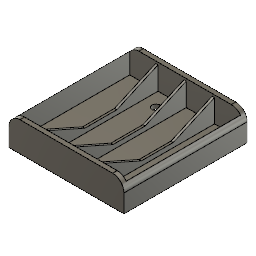
Fusion360_BatteryBox_AAA4 (Autodesk Fusion 360 design; units mm, degrees)
Autodesk Fusion 360 part; units mm, degrees
sketch "スケッチ1" plane through (0, 0, 0) normal (0, 1, 0) x (1, 0, 0)
  line L0 (25.25, -27) -> (-25.25, -27)
  line L1 (-25.25, -27) -> (-25.25, 27)
  line L2 (-25.25, 27) -> (25.25, 27)
  line L3 (25.25, 27) -> (25.25, -27)
  line L4 (25.25, -27) -> (-25.25, 27) construction
  line L5 (-25.25, -27) -> (25.25, 27) construction
  dimension "d1" = 50.5
  dimension "d2" = 54
sketch "スケッチ2" plane through (12.875, 0, 0) normal (1, 0, 0) x (0, 0, -1)
  line L0 (-25, 2) -> (25, 2)
  line L1 (25, 2) -> (25, 12)
  line L2 (25, 12) -> (-25, 12)
  line L3 (-25, 12) -> (-25, 2)
  line L4 (25, 2) -> (7, 2) construction
  line L5 (7, 2) -> (7, 4) construction
  line L6 (7, 4) -> (25, 4) construction
  line L7 (25, 4) -> (25, 2) construction
  line L8 (7, 4) -> (-7, 4)
  line L9 (-7, 4) -> (-7, 12)
  line L10 (-7, 12) -> (7, 12)
  line L11 (7, 12) -> (7, 4)
  dimension "d7" = 18
  dimension "d8" = 2
  dimension "d11" = 14
sketch "スケッチ3" plane through (0, 2, 0) normal (0, 1, 0) x (-1, 0, 0)
  circle A0 centre (-6.1875, 18.4923) radius 1.75
  line L0 (-0.5, -25) -> (-0.5, 25)
  line L1 (-0.5, 25) -> (-11.875, 25)
  line L2 (-11.875, 25) -> (-11.875, -25)
  line L3 (-11.875, -25) -> (-0.5, -25)
  line L4 (-6.1875, 18.4923) -> (6.1875, 18.4923) construction
  line L5 (6.1875, 18.4923) -> (6.1875, -18.4923) construction
  line L6 (6.1875, -18.4923) -> (-6.1875, -18.4923) construction
  line L7 (-6.1875, -18.4923) -> (-6.1875, 18.4923) construction
  circle A1 centre (6.1875, -18.4923) radius 1.75
  dimension "d12" = 12.375
  dimension "d13" = 36.9846
  dimension "d14" = 3.5
  measures "d14" diameter of A1
sketch "スケッチ4" plane through (0, 2, 0) normal (0, 1, 0) x (-1, 0, 0)
  line L0 (-0.5, -25) -> (-0.5, 25)
  line L1 (-0.5, 25) -> (-11.875, 25)
  line L2 (-11.875, 25) -> (-11.875, -25)
  line L3 (-11.875, -25) -> (-0.5, -25)
  line L4 (-11.875, 25) -> (-6.1875, 25) construction
  line L5 (-6.1875, 25) -> (-6.1875, 18.4923) construction
  line L6 (-6.1875, 18.4923) -> (-11.875, 18.4923) construction
  line L7 (-11.875, 18.4923) -> (-11.875, 25) construction
  circle A0 centre (-6.1875, 18.4923) radius 1.75
  dimension "d17" = 5.6875
  dimension "d18" = 6.5077
  dimension "d19" = 3.5
  measures "d19" diameter of A0
sketch "スケッチ5" plane through (0, 2, 0) normal (0, 1, 0) x (-1, 0, 0)
  line L0 (0.5, 25) -> (0.5, -25)
  line L1 (0.5, -25) -> (24.25, -25)
  line L2 (24.25, -25) -> (24.25, 25)
  line L3 (24.25, 25) -> (0.5, 25)
  line L4 (0.5, -25) -> (11.875, -25) construction
  line L5 (11.875, -25) -> (11.875, 25) construction
  line L6 (11.875, 25) -> (0.5, 25) construction
  line L7 (0.5, 25) -> (0.5, -25) construction
  line L8 (11.875, -25) -> (12.875, -25)
  line L9 (12.875, -25) -> (12.875, 25)
  line L10 (12.875, 25) -> (11.875, 25)
  line L11 (11.875, 25) -> (11.875, -25)
  dimension "d20" = 50
  dimension "d23" = 11.375
  dimension "d24" = 1
  dimension "d25" = 50
  measures "d23" distance of origin
sketch "スケッチ6" plane through (0, 2, 0) normal (0, 1, 0) x (-1, 0, 0)
  line L0 (-11.875, 25) -> (-11.875, -25)
  line L1 (-11.875, -25) -> (24.25, -25)
  line L2 (24.25, -25) -> (24.25, 25)
  line L3 (24.25, 25) -> (-11.875, 25)
  line L4 (-11.875, -25) -> (-0.5, -25) construction
  line L5 (-0.5, -25) -> (-0.5, 25) construction
  line L6 (-0.5, 25) -> (-11.875, 25) construction
  line L7 (-11.875, 25) -> (-11.875, -25) construction
  line L8 (-0.5, -25) -> (0.5, -25)
  line L9 (0.5, -25) -> (0.5, 25)
  line L10 (0.5, 25) -> (-0.5, 25)
  line L11 (-0.5, 25) -> (-0.5, -25)
  dimension "d26" = 11.375
  dimension "d29" = 50
  dimension "d30" = 50
  dimension "d31" = 1
  measures "d26" distance of origin
sketch "スケッチ7" plane through (0, 2, 0) normal (0, 1, 0) x (-1, 0, 0)
  line L0 (-24.25, -25) -> (24.25, -25)
  line L1 (24.25, -25) -> (24.25, 25)
  line L2 (24.25, 25) -> (-24.25, 25)
  line L3 (-24.25, 25) -> (-24.25, -25)
  line L4 (-24.25, -25) -> (-12.875, -25) construction
  line L5 (-12.875, -25) -> (-12.875, 25) construction
  line L6 (-12.875, 25) -> (-24.25, 25) construction
  line L7 (-24.25, 25) -> (-24.25, -25) construction
  line L8 (-12.875, -25) -> (-11.875, -25)
  line L9 (-11.875, -25) -> (-11.875, 25)
  line L10 (-11.875, 25) -> (-12.875, 25)
  line L11 (-12.875, 25) -> (-12.875, -25)
  dimension "d38" = 50
  dimension "d39" = 11.375
  dimension "d40" = 50
  dimension "d43" = 1
  measures "d39" distance of origin
sketch "スケッチ8" plane through (12.875, 0, 0) normal (1, 0, 0) x (0, 0, -1)
  line L0 (7, 12) -> (7, 4)
  line L1 (7, 4) -> (-7, 4)
  line L2 (-7, 4) -> (-7, 12)
  line L3 (-7, 12) -> (-25, 12)
  line L4 (-25, 12) -> (-25, 2)
  line L5 (-25, 2) -> (25, 2)
  line L6 (25, 2) -> (25, 12)
  line L7 (25, 12) -> (7, 12)
  line L8 (7, 4) -> (25, 12)
  line L9 (25, 12) -> (7, 12)
  line L10 (7, 12) -> (7, 4)
sketch "スケッチ9" plane through (12.875, 0, 0) normal (1, 0, 0) x (0, 0, -1)
  line L0 (25, 12) -> (7, 4)
  line L1 (7, 4) -> (-7, 4)
  line L2 (-7, 4) -> (-7, 12)
  line L3 (-7, 12) -> (-25, 12)
  line L4 (-25, 12) -> (-25, 2)
  line L5 (-25, 2) -> (25, 2)
  line L6 (25, 2) -> (25, 12)
  line L7 (-7, 12) -> (-7, 4)
  line L8 (-7, 12) -> (-25, 12)
  line L9 (-7, 4) -> (-25, 12)
sketch "スケッチ10" plane through (0, 13, 0) normal (0, 1, 0) x (-1, 0, 0)
  line L0 (20.25, -27) -> (20.25, 27)
  line L1 (20.25, 27) -> (-20.25, 27)
  line L2 (-20.25, 27) -> (-20.25, -27)
  line L3 (-20.25, -27) -> (20.25, -27)
  line L4 (-24.25, 25) -> (24.25, 25)
  line L5 (24.25, 25) -> (24.25, -25)
  line L6 (24.25, -25) -> (-24.25, -25)
  line L7 (-24.25, -25) -> (-24.25, 25)
  line L8 (-24.25, 25) -> (24.25, -25) construction
  line L9 (24.25, 25) -> (-24.25, -25) construction
  dimension "d44" = 48.5
  dimension "d45" = 50
extrude "押し出し1" add sketch "スケッチ1" along normal blind 13
fillet "フィレット1" radius 5 1 edges at (25.25, 13, 0)
fillet "フィレット2" radius 5 1 edges at (-25.25, 13, 0)
extrude "押し出し2" cut sketch "スケッチ10" against normal blind 11 contours L0 L2 L4 L6 | L0 L4 L5 L6 | L2 L4 L6 L7
extrude "押し出し3" add sketch "スケッチ7" along normal blind 10 contours L0 L2 L8 L9 L10 L11
extrude "押し出し4" add sketch "スケッチ6" along normal blind 10 contours L1 L3 L8 L9 L10 L11
extrude "押し出し5" add sketch "スケッチ5" along normal blind 10 contours L1 L3 L8 L9 L10 L11
extrude "押し出し6" cut sketch "スケッチ2" against normal blind 28 contours L2 L8 L9 L10 L11
extrude "押し出し7" cut sketch "スケッチ8" against normal blind 27 contours L0 L7 L8 L9 L10
extrude "押し出し8" cut sketch "スケッチ9" against normal blind 28 contours L2 L3 L7 L8 L9
extrude "押し出し9" cut sketch "スケッチ4" against normal blind 12 contours A0
extrude "押し出し10" cut sketch "スケッチ3" against normal blind 2 contours A1
